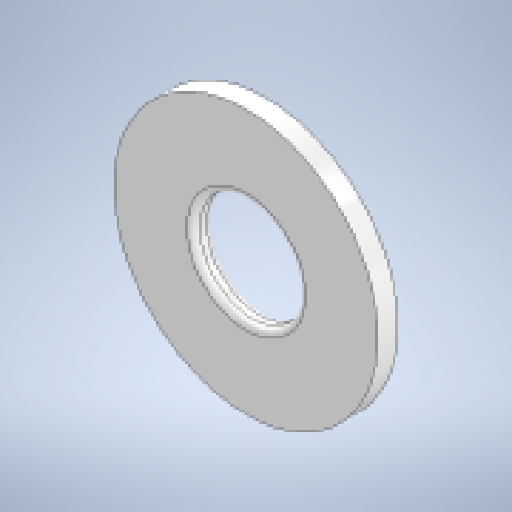
# Autodesk Inventor part: kosiuke
Saved by Autodesk Inventor 2025.1 (Build 291241000, 241)
## iProperties
Created: 2024-09-02
Part Number: kosiuke
Material: ABS プラスチック
Document SubType Name: Modeling
Designer: right
Density: 1.06 g/cm^3
Appearance: 滑らか - 白
Mass: 3.33322 g
Surface Area: 25.9668 cm^2
Volume: 3.14455 cm^3
Author: right
Autodesk Inventor part; units mm, degrees
ref_plane "YZ Plane" through (0, 0, 0) normal (1, 0, 0) x (0, 1, 0)
ref_plane "XZ Plane" through (0, 0, 0) normal (0, 1, 0) x (-1, 0, 0)
sketch "スケッチ1" plane through (0, 0, 0) normal (0, 0, 1) x (1, 0, 0)
  circle A0 centre (0, 0) radius 8 projected
  circle A1 centre (0, 0) radius 20
  point P0 (0, 0)
  dimension "d0" = 40
  constraints: 1 centre point, 1 coincident
  measures "d0" diameter of A1
ref_plane "作業平面1" through (-44.2391, -19.8029, 3) normal (0, 0, -1) x (0.0126013, 0.9999206, 0)
extrude "押し出し1" add sketch "スケッチ1" along normal up to surface (3 mm away)
fillet "フィレット1" radius 1 2 edges at (-8, 0, 0) (-8, 0, 3)
